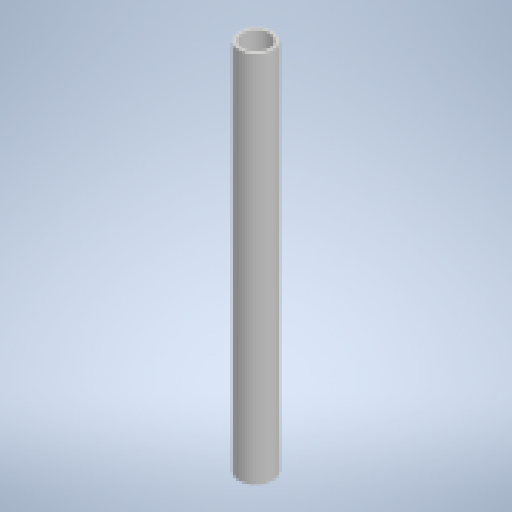
# Autodesk Inventor part: 31000133profil_up(550)
Saved by Autodesk Inventor 2025.2 (Build 292293000, 293)
## iProperties
Category: PARTsolutions
Company: RNA
Created: 2025-06-23
Part Number: 31000133profil_up(550)
Material: Generic
Catalog Web Link: www.cadenas.de
Description: base stand BZB-Accessories
Vendor: RNA
Document SubType Name: Modeling
Designer: psAdmin
Manufacturer: RNA
Mass: 189.099 g
Surface Area: 954.542 cm^2
Volume: 189.099 cm^3
Density: 1 g/cm^3
Appearance: PSOLRGB-175-175-175
PSOL_IDENT_0: {$CADENAS_DATA/23d-libs/rna/bunker/zubehoer/parts/bzb_frofil_up.prj},195 {VTYP=3D},{NB=31000133profi
PSOL_IDENT_1: l_up(550)},{LINA=31000133profil_up(550)},{NN=base stand BZB},{DATE=06.06.2017 07:14:33},{GEOMDATE=01
PSOL_IDENT_2: .02.2017 10:11:00},{VERSION=},{LINEID=200},{WBVAR=H},{WBNUMERIC=H}  {NB=31000133profil_up(550)},{LIN
PSOL_IDENT_3: A=31000133profil_up(550)},{KT=DUMMY},{CNSORDERNO=31000133},{KOMP=Bodenständer BZB 550-900mm BVL3},{T
PSOL_IDENT_4: YP=BVL3},{H=550},{VERS=1},{B=10}
NB: 31000133profil_up(550)
NN: base stand BZB
NT: Accessories
NBSYN: $CNSORDERNO.profil_up($H.)
LINA: 31000133profil_up(550)
CATALOG: Rhein-Nadel-Automation
CNSORDERNO: 31000133
KOMP: Bodenständer BZB 550-900mm BVL3
TYP: BVL3
H: 550
VERS: 1
B: 10
SUPPLIER: RNA
ARTICLENO: 31000133profil_up(550)
BOMINFO: 31000133profil_up(550)
CREATOR: CADENAS GmbH
Title: 31000133profil_up(550)
Author: Cadenas PARTsolutions
Comments: Accessories
Autodesk Inventor part; units mm, degrees
sketch "Sketch_1" plane through (0, 0, 0) normal (0, 1, 0) x (-1, 0, 0)
  circle A0 centre (0, 0) radius 20
  circle A1 centre (0, 0) radius 16
  constraints: 2 centre point
extrude "Extrusion1" add sketch "Sketch_1" along normal blind 450
ref_plane "S2_DOWN_XY" through (0, 0, 0) normal (0, 1, 0) x (1, 0, 0)
ref_plane "S2_DOWN_YZ" through (0, 0, 0) normal (1, 0, 0) x (0, 0, -1)
ref_plane "S2_DOWN_ZX" through (0, 0, 0) normal (0, 0, -1) x (0, 1, 0)
ref_plane "S2_UP_XY" through (0, 418, 0) normal (0, -1, 0) x (1, 0, 0)
ref_plane "S2_UP_YZ" through (0, 418, 0) normal (1, 0, 0) x (0, 0, 1)
ref_plane "S2_UP_ZX" through (0, 418, 0) normal (0, 0, 1) x (0, -1, 0)
body "Solid1"
